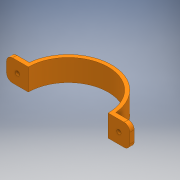
# Autodesk Inventor part: Motor Mount C-Clamp Top
Saved by Autodesk Inventor 2018 (Build 220112000, 112)
## iProperties
Created: 2018-01-11
Part Number: Motor Mount C-Clamp Top
Material: Generic
Document SubType Name: Modeling
Designer: Moochster
Density: 1 g/cm^3
Appearance: Orange
Author: Moochster
Autodesk Inventor part; units mm, degrees
ref_plane "YZ Plane" through (0, 0, 0) normal (1, 0, 0) x (0, 1, 0)
ref_plane "XZ Plane" through (0, 0, 0) normal (0, 1, 0) x (-1, 0, 0)
ref_plane "XY Plane" through (0, 0, 0) normal (0, 0, 1) x (1, 0, 0)
sketch "Sketch1" plane through (0, 0, 0) normal (0, 0, 1) x (1, 0, 0)
  arc A0 (27.54, 0) -> (-27.54, 0) centre (0, 0) ccw
  arc A1 (29.8898, 3) -> (-29.8898, 3) centre (0, 0) ccw
  line L0 (-29.8898, 3) -> (-42.54, 3)
  line L1 (-42.54, 3) -> (-42.54, 0)
  line L2 (-42.54, 0) -> (-27.54, 0)
  line L3 (27.54, 0) -> (42.54, 0)
  line L4 (42.54, 0) -> (42.54, 3)
  line L5 (42.54, 3) -> (29.8898, 3)
  dimension "d0" = 3
  dimension "d1" = 27.54
  dimension "d3" = 2.5
  dimension "d8" = 15
  constraints: 12 end point, 4 horizontal, 4 point on circle, 3 horizontal alignment, 2 centre point, 2 perpendicular, 1 coincident, 1 collinear, 1 concentric
  measures "d0" distance of L3.end L4.end
  measures "d1" radius of A0
  measures "d3" radial gap between concentric circles of A0 A1
  measures "d8" distance of L3.start L3.end
extrude "Extrusion1" add sketch "Sketch1" along normal blind 15
sketch "Sketch2" plane through (-42.54, 0, 0) normal (0, -1, 0) x (1, 0, 0)
  line L0 (0, 15) -> (15, 15) projected
  line L1 (0, 0) -> (0, 15) projected
  point P0 (42.54, 0)
  point P1 (7.5, 7.5)
  point P2 (7.5, 15)
  point P3 (0, 7.5)
  constraints: 2 midpoint, 1 horizontal alignment, 1 vertical alignment
hole "Hole1" at (-35.04, 0, 7.5) direction (0, 1, 0) diameter 3 end through all
mirror "Mirror1" about plane through (0, 0, 0) normal (1, 0, 0) of "Hole1"
fillet "Fillet1" radius 4 4 edges at (-42.54, 1.5, 0) (-42.54, 1.5, 15) (42.54, 1.5, 15) (42.54, 1.5, 0)
body "Solid1"
